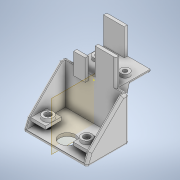
# Autodesk Inventor part: threadedRodMountB
Saved by Autodesk Inventor 2020 (Build 240168000, 168)
## iProperties
Created: 2020-01-08
Part Number: threadedRodMountB
Material: Generic
Document SubType Name: Modeling
Designer: PAB
Density: 1 g/cm^3
Appearance: Default
Author: PAB
Autodesk Inventor part; units mm, degrees
ref_plane "YZ Plane" through (0, 0, 0) normal (1, 0, 0) x (0, 1, 0)
ref_plane "XZ Plane" through (0, 0, 0) normal (0, 1, 0) x (-1, 0, 0)
ref_plane "XY Plane" through (0, 0, 0) normal (0, 0, 1) x (1, 0, 0)
sketch "Sketch1" plane through (0, 0, 0) normal (0, 1, 0) x (-1, 0, 0)
  line L0 (20.5, 16.2) -> (-20.5, 16.2)
  line L1 (-20.5, 16.2) -> (-20.5, -16.2)
  line L2 (-20.5, -16.2) -> (20.5, -16.2)
  line L3 (20.5, -16.2) -> (20.5, 16.2)
  point P0 (0, 0)
  dimension "d0" = 41
  dimension "d1" = 32.4
  constraints: 8 end point, 2 parallel, 1 horizontal, 1 perpendicular
  measures "d0" distance of L2.end L1.end
  measures "d1" distance of L1.end L0.end
extrude "Extrusion1" add sketch "Sketch1" along normal blind 3
sketch "Sketch3" plane through (0, 3, 0) normal (0, 1, 0) x (1, 0, 0)
  line L0 (-20.5, -16.2) -> (20.5, -16.2) projected
  line L1 (-20.5, 16.2) -> (-20.5, -16.2) projected
  line L2 (20.5, -16.2) -> (-20.5, -16.2)
  line L3 (-20.5, -16.2) -> (-20.5, -13.2)
  line L4 (-20.5, -13.2) -> (20.5, -13.2)
  line L5 (20.5, -13.2) -> (20.5, -16.2)
  line L6 (20.5, 16.2) -> (-20.5, 16.2) projected
  line L7 (20.5, 16.2) -> (-20.5, 16.2)
  line L8 (-20.5, 16.2) -> (-20.5, 13.2)
  line L9 (-20.5, 13.2) -> (20.5, 13.2)
  line L10 (20.5, 13.2) -> (20.5, 16.2)
  point P0 (0, 0)
  dimension "d8" = 3
  dimension "d9" = 3
  constraints: 16 end point, 4 parallel, 2 horizontal, 2 perpendicular, 2 point on line
  measures "d8" distance of L2.end L3.end
  measures "d9" distance of L8.end L7.end
extrude "Extrusion3" add sketch "Sketch3" along normal blind 25.4
sketch "Sketch4" plane through (20.5, 0, -16.2) normal (0, 0, -1) x (-1, 0, 0)
  line L0 (41, 3) -> (0, 3) projected
  line L1 (0, 28.4) -> (41, 28.4) projected
  line L2 (0, 3) -> (21.5, 3)
  line L3 (21.5, 3) -> (21.5, 28.4)
  line L4 (21.5, 28.4) -> (0, 28.4)
  line L5 (0, 28.4) -> (0, 3)
  point P0 (20.5, 0)
  dimension "d12" = 21.5
  constraints: 8 end point, 2 parallel, 1 horizontal, 1 perpendicular, 1 point on line
  measures "d12" distance of L4.end L3.end
extrude "Extrusion4" cut sketch "Sketch4" against normal blind 3
sketch "Sketch5" plane through (-20.5, 0, 16.2) normal (0, 0, 1) x (1, 0, 0)
  line L0 (41, 28.4) -> (0, 28.4) projected
  line L1 (19.5, 3) -> (41, 3) projected
  line L2 (0, 28.4) -> (21.5, 28.4)
  line L3 (21.5, 28.4) -> (21.5, 3)
  line L4 (21.5, 3) -> (0, 3)
  line L5 (0, 3) -> (0, 28.4)
  point P0 (20.5, 0)
  dimension "d15" = 21.5
  constraints: 8 end point, 2 parallel, 1 horizontal, 1 perpendicular, 1 point on line
  measures "d15" distance of L3.end L4.end
extrude "Extrusion5" cut sketch "Sketch5" against normal blind 3
sketch "Sketch6" plane through (0, 3, 0) normal (0, 1, 0) x (1, 0, 0)
  circle A0 centre (13, 0) radius 4.25
  circle A1 centre (-13, 0) radius 4.25
  point P0 (0, 0)
  dimension "d20" = 8.5
  dimension "d21" = 8.5
  constraints: 2 centre point
  measures "d20" diameter of A0
  measures "d21" diameter of A1
extrude "Extrusion6" add sketch "Sketch6" along normal blind 3
sketch "Sketch7" plane through (0, 0, 0) normal (0, -1, 0) x (1, 0, 0)
  circle A0 centre (-13, 0) radius 4.25 projected
  circle A1 centre (-13, 0) radius 2
  circle A2 centre (13, 0) radius 4.25 projected
  circle A3 centre (13, 0) radius 2
  point P0 (0, 0)
  dimension "d24" = 4
  dimension "d25" = 4
  constraints: 2 centre point, 2 coincident
  measures "d24" diameter of A1
  measures "d25" diameter of A3
extrude "Extrusion7" cut sketch "Sketch7" against normal blind 6 contours A1 | A3
sketch "Sketch8" plane through (0, 0, 0) normal (0, -1, 0) x (1, 0, 0)
  circle A0 centre (-13, 0) radius 2 projected
  circle A1 centre (-13, 0) radius 3
  circle A2 centre (13, 0) radius 2 projected
  circle A3 centre (13, 0) radius 3
  point P0 (0, 0)
  dimension "d28" = 6
  dimension "d29" = 6
  constraints: 2 centre point, 2 coincident
  measures "d28" diameter of A1
  measures "d29" diameter of A3
extrude "Extrusion8" cut sketch "Sketch8" against normal blind 3 contours A0 | A1 | A2 | A3
sketch "Sketch9" plane through (-20.5, 0, 16.2) normal (0, 0, 1) x (1, 0, 0)
  point P0 (20.5, 0)
sketch "Sketch10" plane through (0, 0, 0) normal (0, -1, 0) x (1, 0, 0)
  line L0 (30, 16.2) -> (-30, 16.2)
  line L1 (-30, 16.2) -> (-30, 13.2)
  line L2 (-30, 13.2) -> (30, 13.2)
  line L3 (30, 13.2) -> (30, 16.2)
  line L4 (-20.5, -16.2) -> (-20.5, 16.2) projected
  line L5 (-20.5, 13.2) -> (-17.5, 13.2)
  line L6 (-17.5, 13.2) -> (-17.5, 3)
  line L7 (-17.5, 3) -> (-20.5, 3)
  line L8 (-20.5, 3) -> (-20.5, 13.2)
  line L9 (-1.5, 13.2) -> (1.5, 13.2)
  line L10 (1.5, 13.2) -> (1.5, 3)
  line L11 (1.5, 3) -> (-1.5, 3)
  line L12 (-1.5, 3) -> (-1.5, 13.2)
  line L13 (20.5, 16.2) -> (20.5, -16.2) projected
  line L14 (20.5, 13.2) -> (17.5, 13.2)
  line L15 (17.5, 13.2) -> (17.5, 3)
  line L16 (17.5, 3) -> (20.5, 3)
  line L17 (20.5, 3) -> (20.5, 13.2)
  point P0 (0, 0)
  dimension "d32" = 60
  dimension "d33" = 3
  dimension "d34" = 3
  dimension "d35" = 3
  dimension "d36" = 3
  constraints: 32 end point, 8 parallel, 7 point on line, 4 horizontal, 4 perpendicular
  measures "d32" distance of L2.end L1.end
  measures "d33" distance of L1.end L0.end
  measures "d34" distance of L6.end L7.end
  measures "d35" distance of L10.end L11.end
  measures "d36" distance of L16.end L15.end
extrude "Extrusion9" add sketch "Sketch10" along normal blind 38.6 and the other way blind 3
sketch "Sketch11" plane through (1, 28.4, 16.2) normal (0, 0, 1) x (1, 0, 0)
  line L0 (19.5, -67) -> (29, -67) projected
  line L1 (-31, -25.4) -> (-31, -67) projected
  line L2 (29, -67) -> (-31, -67)
  line L3 (-31, -67) -> (-31, -64)
  line L4 (-31, -64) -> (29, -64)
  line L5 (29, -64) -> (29, -67)
  line L6 (0, -25.4) -> (-31, -25.4) projected
  line L7 (-31, -64) -> (-28, -64)
  line L8 (-28, -64) -> (-28, -25.4)
  line L9 (-28, -25.4) -> (-31, -25.4)
  line L10 (-31, -25.4) -> (-31, -64)
  line L11 (19.5, -25.4) -> (29, -25.4) projected
  line L12 (29, -64) -> (26, -64)
  line L13 (26, -64) -> (26, -25.4)
  line L14 (26, -25.4) -> (29, -25.4)
  line L15 (29, -25.4) -> (29, -64)
  point P0 (-1, -28.4)
  dimension "d41" = 3
  dimension "d42" = 3
  dimension "d43" = 3
  constraints: 24 end point, 6 parallel, 3 horizontal, 3 perpendicular, 3 point on line
  measures "d41" distance of L2.end L3.end
  measures "d42" distance of L9.end L8.end
  measures "d43" distance of L13.end L14.end
extrude "Extrusion10" add sketch "Sketch11" along normal blind 38
sketch "Sketch12" plane through (1, 28.4, 16.2) normal (0, 0, 1) x (1, 0, 0)
  line L0 (-17.25, -31.4) -> (-6.25, -31.4)
  line L1 (-6.25, -31.4) -> (-6.25, -11.4)
  line L2 (-6.25, -11.4) -> (-17.25, -11.4)
  line L3 (-17.25, -11.4) -> (-17.25, -31.4)
  line L4 (-31, -67) -> (29, -67) projected
  point P0 (-1, -28.4)
  dimension "d46" = 11
  dimension "d47" = 20
  dimension "d48" = 35.6
  constraints: 8 end point, 2 parallel, 1 horizontal, 1 perpendicular
  measures "d46" distance of L2.end L1.end
  measures "d47" distance of L1.end L0.end
  measures "d48" distance between parallel lines of L4 L0
extrude "Extrusion11" add sketch "Sketch12" along normal blind 3
sketch "Sketch13" plane through (27, -35.6, 16.2) normal (-1, 0, 0) x (0, 0, 1)
  line L0 (17.65, 5) -> (32.65, 5)
  line L1 (32.65, 5) -> (32.65, 8)
  line L2 (32.65, 8) -> (17.65, 8)
  line L3 (17.65, 8) -> (17.65, 5)
  point P0 (-16.2, 35.6)
  dimension "d51" = 15
  dimension "d52" = 3
  constraints: 8 end point, 2 parallel, 1 horizontal, 1 perpendicular
  measures "d51" distance of L2.end L1.end
  measures "d52" distance of L1.end L0.end
extrude "Extrusion12" add sketch "Sketch13" along normal blind 14
sketch "Sketch14" plane through (27, -27.6, 48.85) normal (0, 1, 0) x (1, 0, 0)
  circle A0 centre (-8.75, 7.5) radius 5
  circle A1 centre (-8.75, 7.5) radius 3
  point P0 (-27, 48.85)
  dimension "d55" = 10
  dimension "d56" = 6
  constraints: 2 centre point, 1 coincident
  measures "d55" diameter of A0
  measures "d56" diameter of A1
extrude "Extrusion13" add sketch "Sketch14" along normal blind 3
sketch "Sketch15" plane through (18.25, -27.6, 41.35) normal (0, 1, 0) x (1, 0, 0)
  circle A0 centre (0, 0) radius 3 projected
  circle A1 centre (0, 0) radius 2
  point P0 (-18.25, 41.35)
  dimension "d59" = 4
  constraints: 1 centre point, 1 coincident
  measures "d59" diameter of A1
extrude "Extrusion14" cut sketch "Sketch15" against normal blind 20 contours A1
ref_plane "Work Plane1" through (0, -38.6, 13.2) normal (1, 0, 0) x (0, 0, -1)
mirror "Mirror1" about plane through (0, -38.6, 13.2) normal (1, 0, 0) of "Extrusion14", "Extrusion13", "Extrusion12"
sketch "Sketch16" plane through (-27, -35.6, 16.2) normal (0, 1, 0) x (1, 0, 0)
  circle A0 centre (27, -25.15) radius 7.5
  point P0 (27, 16.2)
  dimension "d63" = 15
  constraints: 1 centre point
  measures "d63" diameter of A0
extrude "Extrusion15" cut sketch "Sketch16" against normal blind 20
sketch "Sketch17" plane through (-30, -38.6, 13.2) normal (-1, 0, 0) x (0, 0, 1)
  line L0 (-10.2, 38.6) -> (-10.2, 0) projected
  line L1 (-10.2, 38.6) -> (-10.2, 0)
  line L2 (0, 0) -> (-10.2, 0) projected
  line L3 (-10.2, 0) -> (0, 0)
  line L4 (0, 0) -> (-10.2, 38.6)
  line L5 (0, 41.6) -> (41, 41.6) projected
  line L6 (6, 41.6) -> (36.6, 11)
  line L7 (6, 41.6) -> (49.2749, 41.6) construction
  line L8 (41, 0) -> (41, 41.6) projected
  line L9 (36.6, 11) -> (41, 0)
  line L10 (41, 0) -> (41, 41.6)
  line L11 (41, 41.6) -> (6, 41.6)
  point P0 (-13.2, 38.6)
  dimension "d66" = 45
  constraints: 16 end point, 3 collinear, 1 equal length, 1 horizontal, 1 perpendicular, 1 point on line
  measures "d66" angle of L6 L7
extrude "Extrusion16" cut sketch "Sketch17" against normal blind 60
fillet "Fillet1" radius 2 5 edges at (-20.5, 14.2, -16.2) (-20.5, 0, -6.6) (0, 0, -16.2) (20.5, 0, -6.6) (20.5, 15.7, 16.2)
fillet "Fillet2" radius 1 8 edges at (20.5, 1, 2.7358) (20.5, -19.3, 8.1) (17.5, -19.3, 8.1) (1.5, -19.3, 8.1) (-1.5, -19.3, 8.1) (-17.5, -19.3, 8.1) (-20.5, 1, 2.7358) (-20.5, -19.3, 8.1)
fillet "Fillet3" radius 2 9 edges at (30, -38.6, 33.7) (0, -38.6, 54.2) (-30, -38.6, 33.7) (-18, -38.6, 13.2) (-9.5, -38.6, 13.2) (-1, -38.6, 13.2) (1, -38.6, 13.2) (9.5, -38.6, 13.2) (18, -38.6, 13.2)
fillet "Fillet4" radius 2 8 edges at (-29.4142, -38.0142, 13.2) (-30, -16.8, 13.2) (-24.25, -38.6, 13.2) (-20, -38.6, 13.2) (29.4142, -38.0142, 13.2) (30, -16.8, 13.2) (24.25, -38.6, 13.2) (20, -38.6, 13.2)
fillet "Fillet5" radius 2 14 edges at (-30, -12.3, 34.5) (-30, -36.2218, 53.2098) (-29.4142, -38.0142, 52.6601) (-30, -31.7286, 51.4514) (30, -36.2218, 53.2098) (29.4142, -38.0142, 52.6601) (30, -31.7286, 51.4514) (30, -12.3, 34.5) (29.4142, 3, 13.7858) (24.25, 3, 13.2) (30, 3, 17.2) (-29.4142, 3, 13.7858) (-30, 3, 17.2) (-24.25, 3, 13.2)
body "Solid1"
